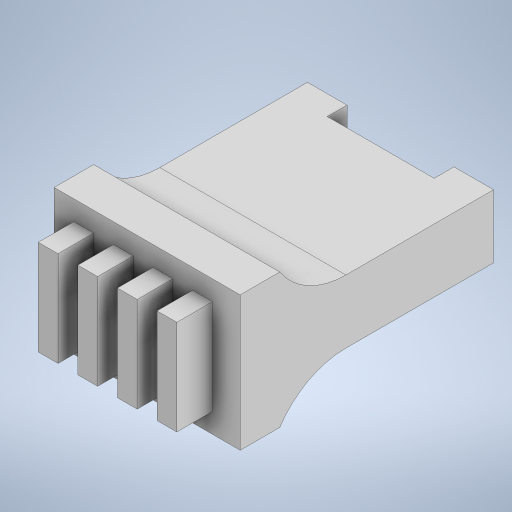
# Autodesk Inventor part: wlacznik_2
Saved by Autodesk Inventor 2023 (Build 270158000, 158)
## iProperties
Created: 2023-08-22
Part Number: wlacznik_2
Material: Ogólny
Document SubType Name: Modeling
Designer: Kamil
Density: 1 g/cm^3
Appearance: Domyślna
Author: Kamil
Autodesk Inventor part; units mm, degrees
ref_plane "YZ Plane" through (0, 0, 0) normal (1, 0, 0) x (0, 1, 0)
ref_plane "XZ Plane" through (0, 0, 0) normal (0, 1, 0) x (-1, 0, 0)
sketch "Szkic1" plane through (0, 0, 0) normal (0, 0, 1) x (1, 0, 0)
  line L0 (2.7, 2.2) -> (2.7, 0.4) projected
  line L1 (5, 0.4) -> (5, 2.2) projected
  line L2 (5, 2.2) -> (5, 2.6) projected
  line L3 (2.7, 2.6) -> (2.7, 2.2) projected
  line L4 (2.7, 0.4) -> (2.7, 0) projected
  line L5 (5, 0) -> (5, 0.4) projected
  line L6 (2.7, 0) -> (5, 0) projected
  line L7 (5, 2.6) -> (2.7, 2.6) projected
  line L8 (2.5, -0.2) -> (2.5, 0.4)
  line L9 (2.5, 0.4) -> (2.5, 2.2)
  line L10 (2.5, 2.2) -> (2.5, 2.8)
  line L11 (2.5, 2.8) -> (5.2, 2.8)
  line L12 (5.2, 2.8) -> (5.2, 2.2)
  line L13 (5.2, 2.2) -> (5.2, 0.4)
  line L14 (5.2, 0.4) -> (5.2, -0.2)
  line L15 (5.2, -0.2) -> (2.5, -0.2)
  line L16 (2.7, 0) -> (2.7, 2.6) projected
  line L17 (0, 2.6) -> (2.7, 2.6) projected
  line L18 (0, 0) -> (0, 2.6) projected
  line L19 (0, 0) -> (2.7, 0) projected
  line L20 (5, 2.6) -> (5, 0) projected
  line L21 (5, 0) -> (10, 0) projected
  line L22 (10, 0) -> (10, 2.6) projected
  line L23 (5, 2.6) -> (10, 2.6) projected
  line L24 (2.5, 0) -> (1.5, 0)
  line L25 (1.5, 0) -> (1.5, 2.6)
  line L26 (1.5, 2.6) -> (2.5, 2.6)
  line L27 (2.5, 2.6) -> (2.5, 0)
  line L28 (5.2, 0) -> (6.2, 0)
  line L29 (6.2, 0) -> (6.2, 2.6)
  line L30 (6.2, 2.6) -> (5.2, 2.6)
  line L31 (5.2, 2.6) -> (5.2, 0)
  dimension "d0" = 0.2
  dimension "d1" = 1
  dimension "d2" = 1
  constraints: 32 end point, 6 point on line, 4 parallel, 2 horizontal, 2 perpendicular, 7 other
  measures "d0" distance between parallel lines of L4 L8
  measures "d1" distance of L25.end L26.end
  measures "d2" distance of L30.end L29.end
extrude "Wyciągnięcie proste1" add sketch "Szkic1" along normal blind 0.5 contours L10 L9 L8 L19 L25 L17 | L23 L29 L21 L14 L13 L12
sketch "Szkic2" plane through (0, 0, 0.5) normal (0, 0, 1) x (1, 0, 0)
  line L0 (1.5, 0) -> (2.5, 0) projected
  line L1 (2.5, 0) -> (2.5, 2.6) projected
  line L2 (2.5, 2.6) -> (1.5, 2.6) projected
  line L3 (1.5, 2.6) -> (1.5, 0) projected
  line L4 (6.2, 2.6) -> (5.2, 2.6) projected
  line L5 (5.2, 2.6) -> (5.2, 0) projected
  line L6 (5.2, 0) -> (6.2, 0) projected
  line L7 (6.2, 0) -> (6.2, 2.6) projected
  line L8 (1.5, 2.6) -> (6.2, 2.6)
  line L9 (6.2, 2.6) -> (6.2, 0)
  line L10 (6.2, 0) -> (1.5, 0)
  line L11 (1.5, 0) -> (1.5, 2.6)
  point P0 (0, 0)
  constraints: 8 end point, 2 parallel, 1 horizontal, 1 perpendicular
ref_plane "Płaszczyzna konstrukcyjna1" through (-1, -0.5, 6.4) normal (0, 0, -1) x (0, 1, 0)
extrude "Wyciągnięcie proste2" add sketch "Szkic2" along normal up to surface (5.9 mm away)
sketch "Szkic3" plane through (1.5, 0, 6.4) normal (0, 0, 1) x (1, 0, 0)
  line L0 (9.5, 3.1) -> (-2.5, 3.1) projected
  line L1 (-2.5, 3.1) -> (-2.5, -0.5) projected
  line L2 (-2.5, -0.5) -> (9.5, -0.5) projected
  line L3 (9.5, -0.5) -> (9.5, 3.1) projected
  line L4 (0, 2.6) -> (0, 0) projected
  line L5 (0, 0) -> (4.7, 0) projected
  line L6 (4.7, 0) -> (4.7, 2.6) projected
  line L7 (4.7, 2.6) -> (0, 2.6) projected
  line L8 (0, 3.1) -> (4.7, 3.1)
  line L9 (4.7, 3.1) -> (4.7, -0.5)
  line L10 (4.7, -0.5) -> (0, -0.5)
  line L11 (0, -0.5) -> (0, 3.1)
  line L12 (-2.4, 3) -> (9.4, 3)
  line L13 (9.4, 3) -> (9.4, -0.4)
  line L14 (9.4, -0.4) -> (-2.4, -0.4)
  line L15 (-2.4, -0.4) -> (-2.4, 3)
  point P0 (-1.5, 0)
  point P1 (4.7, 3)
  point P2 (0, 3)
  point P3 (0, -0.4)
  point P4 (4.7, -0.4)
  dimension "d7" = 0.1
  constraints: 16 end point, 2 parallel, 2 point on line, 1 horizontal, 1 perpendicular, 3 other
  measures "d7" distance between parallel lines of L0 L12
extrude "Wyciągnięcie proste3" add sketch "Szkic3" against normal blind 1 contours L9 L7 L11 L12 | L6 L5 L4 L7 | L14 L11 L5 L9
sketch "Szkic4" plane through (1.5, -0.4, 6.4) normal (0, 0, 1) x (1, 0, 0)
  line L0 (-2.2, 3.2) -> (9.2, 3.2) projected
  line L1 (9.2, 0.2) -> (-2.2, 0.2) projected
  line L2 (-2.2, 0.2) -> (-2.2, 3.2) projected
  line L3 (9.2, 3.2) -> (9.2, 0.2) projected
  line L4 (0, 3.4) -> (0, 0) projected
  line L5 (0, 0) -> (4.7, 0) projected
  line L6 (4.7, 0) -> (4.7, 3.4) projected
  line L7 (4.7, 3.4) -> (0, 3.4) projected
  line L8 (0.5, 0.5) -> (0.5, 2.9)
  line L9 (0.5, 2.9) -> (4.2, 2.9)
  line L10 (4.2, 2.9) -> (4.2, 0.5)
  line L11 (4.2, 0.5) -> (0.5, 0.5)
  line L12 (1, 0.4) -> (1, 3) projected
  line L13 (0.5, 2.9) -> (1, 2.9)
  line L14 (1, 2.9) -> (1, 0.5)
  line L15 (1, 0.5) -> (0.5, 0.5)
  line L16 (0.5, 0.5) -> (0.5, 2.9)
  line L17 (1.5, 2.9) -> (1.5, 0.5)
  line L18 (2, 2.9) -> (2, 0.5)
  line L19 (2.5, 2.9) -> (2.5, 0.5)
  line L20 (3, 2.9) -> (3, 0.5)
  line L21 (3.5, 2.9) -> (3.5, 0.5)
  line L22 (4, 2.9) -> (4, 0.5)
  point P0 (-1.5, 0.4)
  point P1 (4, 0.5)
  point P2 (4, 2.9)
  point P3 (3.5, 2.9)
  point P4 (3.5, 0.5)
  point P5 (3, 0.5)
  point P6 (3, 2.9)
  point P7 (2.5, 0.5)
  point P8 (2, 0.5)
  point P9 (1.5, 2.9)
  point P10 (1.5, 0.5)
  point P11 (1, 2.9)
  dimension "d10" = 0.5
  dimension "d13" = 0.5
  constraints: 28 end point, 2 horizontal, 2 parallel, 2 point on line, 1 perpendicular, 21 other
  measures "d10" distance between parallel lines of L4 L8
  measures "d13" distance of L13.end L17.start
extrude "Wyciągnięcie proste4" add sketch "Szkic4" along normal blind 0.9 contours L8 L9 L12 L11 | L17 L9 L18 L11 | L19 L9 L20 L11 | L21 L9 L22 L11
sketch "Szkic5" plane through (1.5, 0, 0) normal (0, -1, 0) x (1, 0, 0)
  line L0 (4.7, 5.4) -> (0, 5.4) projected
  line L1 (0, 0) -> (0, 5.4) projected
  line L2 (0, 0) -> (1, 0) projected
  line L3 (1, 0) -> (1, 0.5) projected
  line L4 (1, 0.5) -> (3.7, 0.5) projected
  line L5 (3.7, 0) -> (3.7, 0.5) projected
  line L6 (3.7, 0) -> (4.7, 0) projected
  line L7 (4.7, 0) -> (4.7, 5.4) projected
  point P0 (-1.5, 0)
extrude "Wyciągnięcie proste5" cut sketch "Szkic5" against normal blind 0.5
sketch "Szkic6" plane through (5.2, 2.6, 0) normal (0, 1, 0) x (1, 0, 0)
  line L0 (-3.7, -5.4) -> (1, -5.4) projected
  line L1 (1, 0) -> (1, -5.4) projected
  line L2 (1, 0) -> (0, 0) projected
  line L3 (0, 0) -> (0, -0.5) projected
  line L4 (0, -0.5) -> (-2.7, -0.5) projected
  line L5 (-2.7, 0) -> (-2.7, -0.5) projected
  line L6 (-2.7, 0) -> (-3.7, 0) projected
  line L7 (-3.7, 0) -> (-3.7, -5.4) projected
  point P0 (-5.2, 0)
extrude "Wyciągnięcie proste6" cut sketch "Szkic6" against normal blind 0.5
fillet "Zaokrąglenie1" radius 2 2 edges at (3.85, 2.1, 5.4) (3.85, 0.5, 5.4)
